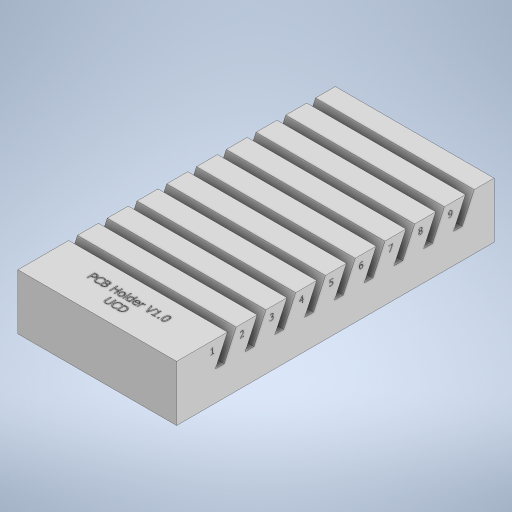
# Autodesk Inventor part: Part1
Saved by Autodesk Inventor 2024 (Build 280153000, 153)
## iProperties
Created: 2024-10-10
Part Number: Part1
Material: Generic
Document SubType Name: Modeling
Designer: Kemper Room 121
Density: 1 g/cm^3
Appearance: Default
Author: Kemper Room 121
Autodesk Inventor part; units mm, degrees
ref_plane "YZ Plane" through (0, 0, 0) normal (1, 0, 0) x (0, 1, 0)
ref_plane "XZ Plane" through (0, 0, 0) normal (0, 1, 0) x (-1, 0, 0)
sketch "Sketch1" plane through (0, 0, 0) normal (1, 0, 0) x (0, 1, 0)
  line L0 (0, 0) -> (10, 0)
  line L1 (10, 0) -> (28, 0)
  line L2 (28, 0) -> (28, -160)
  line L3 (28, -160) -> (0, -160)
  line L4 (0, -160) -> (0, 0)
  dimension "d0" = 10
  dimension "d1" = 18
  dimension "d2" = 160
  constraints: 10 end point, 3 perpendicular, 1 horizontal, 1 point on line
  measures "d0" distance of L0.start L0.end
  measures "d1" distance of L0.end L1.end
  measures "d2" distance of L1.end L2.end
extrude "Extrusion1" add sketch "Sketch1" along normal blind 80
sketch "Sketch2" plane through (80, 0, 0) normal (1, 0, 0) x (0, 0, -1)
  line L0 (0, 28) -> (0, 0) projected
  line L1 (0, 0) -> (0, 5)
  line L2 (160, 0) -> (160, 28) projected
  line L3 (160, 28) -> (0, 28) projected
  line L4 (0, 28) -> (0, 0) projected
  line L5 (0, 0) -> (160, 0) projected
  line L6 (0, 5) -> (160, 5)
  line L7 (160, 5) -> (160, 28)
  line L8 (160, 28) -> (0, 28)
  line L9 (0, 28) -> (0, 5)
  line L10 (160, 28) -> (0, 28) projected
  line L11 (150, 28) -> (139.2749, 5)
  line L12 (145.5865, 28) -> (134.8614, 5)
  line L13 (135, 28) -> (124.2749, 5)
  line L14 (130.5865, 28) -> (119.8614, 5)
  line L15 (120, 28) -> (109.2749, 5)
  line L16 (115.5865, 28) -> (104.8614, 5)
  line L17 (105, 28) -> (94.2749, 5)
  line L18 (100.5865, 28) -> (89.8614, 5)
  line L19 (90, 28) -> (79.2749, 5)
  line L20 (85.5865, 28) -> (74.8614, 5)
  line L21 (75, 28) -> (64.2749, 5)
  line L22 (70.5865, 28) -> (59.8614, 5)
  line L23 (60, 28) -> (49.2749, 5)
  line L24 (55.5865, 28) -> (44.8614, 5)
  line L25 (45, 28) -> (34.2749, 5)
  line L26 (40.5865, 28) -> (29.8614, 5)
  line L27 (30, 28) -> (19.2749, 5)
  line L28 (25.5865, 28) -> (14.8614, 5)
  line L29 (15, 28) -> (4.2749, 5)
  line L30 (10.5865, 28) -> (-0.1386, 5)
  line L31 (10.8067, 29.0831) -> (14.4923, 29.0831) construction
  line L32 (14.4923, 29.0831) -> (14.4923, 25.1764) construction
  line L33 (14.4923, 25.1764) -> (10.8067, 25.1764) construction
  line L34 (10.8067, 25.1764) -> (10.8067, 29.0831) construction
  point P0 (40.5865, 28)
  point P1 (29.8614, 5)
  point P2 (34.2749, 5)
  point P3 (45, 28)
  point P4 (55.5865, 28)
  point P5 (44.8614, 5)
  point P6 (49.2749, 5)
  point P7 (60, 28)
  point P8 (70.5865, 28)
  point P9 (59.8614, 5)
  point P10 (64.2749, 5)
  point P11 (75, 28)
  point P12 (85.5865, 28)
  point P13 (74.8614, 5)
  point P14 (79.2749, 5)
  point P15 (90, 28)
  point P16 (100.5865, 28)
  point P17 (89.8614, 5)
  point P18 (94.2749, 5)
  point P19 (105, 28)
  point P20 (115.5865, 28)
  point P21 (104.8614, 5)
  point P22 (109.2749, 5)
  point P23 (119.8614, 5)
  point P24 (124.2749, 5)
  point P25 (0, 7.2972)
  point P26 (0, 7.2972)
  point P27 (25.5865, 28)
  point P28 (14.8614, 5)
  point P29 (19.2749, 5)
  point P30 (30, 28)
  dimension "d5" = 5
  dimension "d6" = 4
  dimension "d7" = 10
  dimension "d10" = 15
  dimension "d15" = 65
  constraints: 48 end point, 36 horizontal alignment, 20 parallel, 3 point on line, 1 horizontal, 1 vertical, 8 other
  measures "d5" distance of L0.end L1.end
  measures "d6" distance between parallel lines of L12 L11
  measures "d7" distance of L2.end L11.start
  measures "d10" distance of L11.start L13.start
  measures "d15" angle to the sketch x axis of L11
extrude "Extrusion2" cut sketch "Sketch2" against normal through all contours L28 L3 L27 L6 | L6 L12 L3 L11 | L26 L3 L25 L6 | L6 L14 L3 L13 | L24 L3 L23 L6 | L6 L16 L3 L15 | L22 L3 L21 L6 | L6 L18 L3 L17 | L20 L3 L19 L6
sketch "Sketch3" plane through (80, 0, 0) normal (1, 0, 0) x (0, 0, -1)
  line L0 (16.8059, 25) -> (19.0865, 25) construction
  line L1 (19.0865, 25) -> (19.0865, 23.4511) construction
  line L2 (19.0865, 23.4511) -> (16.8059, 23.4511) construction
  line L3 (16.8059, 23.4511) -> (16.8059, 25) construction
  line L4 (31.8059, 25) -> (34.0865, 25) construction
  line L5 (34.0865, 25) -> (34.0865, 23.6664) construction
  line L6 (34.0865, 23.6664) -> (31.8059, 23.6664) construction
  line L7 (31.8059, 23.6664) -> (31.8059, 25) construction
  line L8 (46.8059, 21.9511) -> (46.8059, 25) construction
  line L9 (46.8059, 25) -> (49.0865, 25) construction
  line L10 (49.0865, 25) -> (49.0865, 21.9511) construction
  line L11 (49.0865, 21.9511) -> (46.8059, 21.9511) construction
  line L12 (61.8059, 21.9511) -> (61.8059, 25) construction
  line L13 (61.8059, 25) -> (64.0865, 25) construction
  line L14 (64.0865, 25) -> (64.0865, 21.9511) construction
  line L15 (64.0865, 21.9511) -> (61.8059, 21.9511) construction
  line L16 (76.8059, 21.9511) -> (76.8059, 25) construction
  line L17 (76.8059, 25) -> (79.0865, 25) construction
  line L18 (79.0865, 25) -> (79.0865, 21.9511) construction
  line L19 (79.0865, 21.9511) -> (76.8059, 21.9511) construction
  line L20 (91.8059, 21.9511) -> (91.8059, 25) construction
  line L21 (91.8059, 25) -> (94.0865, 25) construction
  line L22 (94.0865, 25) -> (94.0865, 21.9511) construction
  line L23 (94.0865, 21.9511) -> (91.8059, 21.9511) construction
  line L24 (106.8059, 21.9511) -> (106.8059, 25) construction
  line L25 (106.8059, 25) -> (109.0865, 25) construction
  line L26 (109.0865, 25) -> (109.0865, 21.9511) construction
  line L27 (109.0865, 21.9511) -> (106.8059, 21.9511) construction
  line L28 (121.8059, 21.9511) -> (121.8059, 25) construction
  line L29 (121.8059, 25) -> (124.0865, 25) construction
  line L30 (124.0865, 25) -> (124.0865, 21.9511) construction
  line L31 (124.0865, 21.9511) -> (121.8059, 21.9511) construction
  line L32 (70.5865, 28) -> (0, 28) projected
  line L33 (160, 28) -> (150, 28) projected
  line L34 (70.5865, 28) -> (0, 28) projected
  line L35 (85.5865, 28) -> (75, 28) projected
  line L36 (100.5865, 28) -> (90, 28) projected
  line L37 (115.5865, 28) -> (105, 28) projected
  line L38 (130.5865, 28) -> (120, 28) projected
  line L39 (145.5865, 28) -> (135, 28) projected
  line L40 (0, 28) -> (0, 0) projected
  line L41 (104.8614, 5) -> (115.5865, 28) projected
  line L42 (115.5865, 28) -> (105, 28) projected
  line L43 (105, 28) -> (94.2749, 5) projected
  line L44 (94.2749, 5) -> (89.8614, 5) projected
  line L45 (89.8614, 5) -> (100.5865, 28) projected
  line L46 (100.5865, 28) -> (90, 28) projected
  line L47 (90, 28) -> (79.2749, 5) projected
  line L48 (79.2749, 5) -> (74.8614, 5) projected
  line L49 (74.8614, 5) -> (85.5865, 28) projected
  line L50 (85.5865, 28) -> (75, 28) projected
  line L51 (75, 28) -> (64.2749, 5) projected
  line L52 (64.2749, 5) -> (59.8614, 5) projected
  line L53 (59.8614, 5) -> (70.5865, 28) projected
  line L54 (70.5865, 28) -> (60, 28) projected
  line L55 (60, 28) -> (49.2749, 5) projected
  line L56 (49.2749, 5) -> (44.8614, 5) projected
  line L57 (44.8614, 5) -> (55.5865, 28) projected
  line L58 (55.5865, 28) -> (45, 28) projected
  line L59 (45, 28) -> (34.2749, 5) projected
  line L60 (34.2749, 5) -> (29.8614, 5) projected
  line L61 (29.8614, 5) -> (40.5865, 28) projected
  line L62 (40.5865, 28) -> (30, 28) projected
  line L63 (30, 28) -> (19.2749, 5) projected
  line L64 (19.2749, 5) -> (14.8614, 5) projected
  line L65 (14.8614, 5) -> (25.5865, 28) projected
  line L66 (25.5865, 28) -> (0, 28) projected
  line L67 (0, 28) -> (0, 0) projected
  line L68 (0, 0) -> (160, 0) projected
  line L69 (160, 0) -> (160, 28) projected
  line L70 (160, 28) -> (150, 28) projected
  line L71 (150, 28) -> (139.2749, 5) projected
  line L72 (139.2749, 5) -> (134.8614, 5) projected
  line L73 (134.8614, 5) -> (145.5865, 28) projected
  line L74 (145.5865, 28) -> (135, 28) projected
  line L75 (135, 28) -> (124.2749, 5) projected
  line L76 (124.2749, 5) -> (119.8614, 5) projected
  line L77 (119.8614, 5) -> (130.5865, 28) projected
  line L78 (130.5865, 28) -> (120, 28) projected
  line L79 (120, 28) -> (109.2749, 5) projected
  line L80 (109.2749, 5) -> (104.8614, 5) projected
  line L81 (136.8059, 21.9511) -> (136.8059, 25) construction
  line L82 (136.8059, 25) -> (139.0865, 25) construction
  line L83 (139.0865, 25) -> (139.0865, 21.9511) construction
  line L84 (139.0865, 21.9511) -> (136.8059, 21.9511) construction
  line L85 (18.7548, 21.9421) -> (17.2678, 21.9421)
  line L86 (17.2678, 21.9421) -> (17.2678, 22.2533)
  line L87 (17.2678, 22.2533) -> (17.8211, 22.2533)
  line L88 (17.8211, 22.2533) -> (17.8211, 24.296)
  line L89 (17.8211, 24.296) -> (17.2678, 24.296)
  line L90 (17.2678, 24.296) -> (17.2678, 24.5752)
  spline S0 degree 2 poles (17.2678, 24.5752) (17.5815, 24.5752) (17.8779, 24.753) (17.8977, 25) knots 0 0 0 1 2 2 2
  line L91 (17.8977, 25) -> (18.2139, 25)
  line L92 (18.2139, 25) -> (18.2139, 22.2533)
  line L93 (18.2139, 22.2533) -> (18.7548, 22.2533)
  line L94 (18.7548, 22.2533) -> (18.7548, 21.9421)
  line L95 (33.9079, 21.8878) -> (32.0282, 21.8878)
  line L96 (32.0282, 21.8878) -> (32.0282, 22.32)
  spline S1 degree 2 poles (32.0282, 22.32) (32.2308, 22.5102) (32.5914, 22.8634) (32.7643, 23.0536) knots 0 0 0 1 2 2 2
  spline S2 degree 2 poles (32.7643, 23.0536) (33.1126, 23.4365) (33.367, 23.8959) (33.367, 24.1404) knots 0 0 0 1 2 2 2
  spline S3 degree 2 poles (33.367, 24.1404) (33.367, 24.2689) (33.288, 24.4615) (33.2163, 24.5233) knots 0 0 0 1 2 2 2
  spline S4 degree 2 poles (33.2163, 24.5233) (33.1447, 24.585) (32.957, 24.6468) (32.8434, 24.6468) knots 0 0 0 1 2 2 2
  spline S5 degree 2 poles (32.8434, 24.6468) (32.7347, 24.6468) (32.5124, 24.5924) (32.4111, 24.5505) knots 0 0 0 1 2 2 2
  spline S6 degree 2 poles (32.4111, 24.5505) (32.3247, 24.5159) (32.1641, 24.4171) (32.1147, 24.3825) knots 0 0 0 1 2 2 2
  line L97 (32.1147, 24.3825) -> (32.0925, 24.3825)
  line L98 (32.0925, 24.3825) -> (32.0925, 24.8172)
  spline S7 degree 2 poles (32.0925, 24.8172) (32.2184, 24.879) (32.6705, 25) (32.873, 25) knots 0 0 0 1 2 2 2
  spline S8 degree 2 poles (32.873, 25) (33.3003, 25) (33.782, 24.548) (33.782, 24.1627) knots 0 0 0 1 2 2 2
  spline S9 degree 2 poles (33.782, 24.1627) (33.782, 23.9824) (33.698, 23.681) (33.6239, 23.5526) knots 0 0 0 1 2 2 2
  spline S10 degree 2 poles (33.6239, 23.5526) (33.5498, 23.4192) (33.3349, 23.1574) (33.2163, 23.0314) knots 0 0 0 1 2 2 2
  spline S11 degree 2 poles (33.2163, 23.0314) (33.0237, 22.8214) (32.5519, 22.3719) (32.4111, 22.241) knots 0 0 0 1 2 2 2
  line L99 (32.4111, 22.241) -> (33.9079, 22.241)
  line L100 (33.9079, 22.241) -> (33.9079, 21.8878)
  spline S12 degree 2 poles (47.8508, 24.6468) (47.7396, 24.6468) (47.5198, 24.5924) (47.4136, 24.5505) knots 0 0 0 1 2 2 2
  spline S13 degree 2 poles (47.4136, 24.5505) (47.3148, 24.5085) (47.169, 24.4195) (47.1122, 24.38) knots 0 0 0 1 2 2 2
  line L101 (47.1122, 24.38) -> (47.0875, 24.38)
  line L102 (47.0875, 24.38) -> (47.0875, 24.8123)
  spline S14 degree 2 poles (47.0875, 24.8123) (47.2209, 24.8839) (47.6779, 25) (47.8829, 25) knots 0 0 0 1 2 2 2
  spline S15 degree 2 poles (47.8829, 25) (48.0904, 25) (48.3991, 24.916) (48.5251, 24.8271) knots 0 0 0 1 2 2 2
  spline S16 degree 2 poles (48.5251, 24.8271) (48.6585, 24.7308) (48.7968, 24.4517) (48.7968, 24.2639) knots 0 0 0 1 2 2 2
  spline S17 degree 2 poles (48.7968, 24.2639) (48.7968, 24.012) (48.4658, 23.6316) (48.2336, 23.5822) knots 0 0 0 1 2 2 2
  line L103 (48.2336, 23.5822) -> (48.2336, 23.5526)
  spline S18 degree 2 poles (48.2336, 23.5526) (48.3299, 23.5328) (48.5498, 23.4439) (48.6436, 23.355) knots 0 0 0 1 2 2 2
  spline S19 degree 2 poles (48.6436, 23.355) (48.7375, 23.2685) (48.8561, 22.9919) (48.8561, 22.7918) knots 0 0 0 1 2 2 2
  spline S20 degree 2 poles (48.8561, 22.7918) (48.8561, 22.5868) (48.7153, 22.2385) (48.5868, 22.1051) knots 0 0 0 1 2 2 2
  spline S21 degree 2 poles (48.5868, 22.1051) (48.4534, 21.9668) (48.0755, 21.8236) (47.8359, 21.8236) knots 0 0 0 1 2 2 2
  spline S22 degree 2 poles (47.8359, 21.8236) (47.6062, 21.8236) (47.1567, 21.9347) (47.0035, 22.0113) knots 0 0 0 1 2 2 2
  line L104 (47.0035, 22.0113) -> (47.0035, 22.4435)
  line L105 (47.0035, 22.4435) -> (47.0332, 22.4435)
  spline S23 degree 2 poles (47.0332, 22.4435) (47.1616, 22.3497) (47.5964, 22.1768) (47.8112, 22.1768) knots 0 0 0 1 2 2 2
  spline S24 degree 2 poles (47.8112, 22.1768) (47.9372, 22.1768) (48.1892, 22.2558) (48.2731, 22.3472) knots 0 0 0 1 2 2 2
  spline S25 degree 2 poles (48.2731, 22.3472) (48.3546, 22.4386) (48.4411, 22.656) (48.4411, 22.8214) knots 0 0 0 1 2 2 2
  spline S26 degree 2 poles (48.4411, 22.8214) (48.4411, 22.9869) (48.3448, 23.2018) (48.2583, 23.2636) knots 0 0 0 1 2 2 2
  spline S27 degree 2 poles (48.2583, 23.2636) (48.1719, 23.3253) (47.9372, 23.3723) (47.7989, 23.3723) knots 0 0 0 1 2 2 2
  line L106 (47.7989, 23.3723) -> (47.626, 23.3723)
  line L107 (47.626, 23.3723) -> (47.626, 23.7107)
  line L108 (47.626, 23.7107) -> (47.7618, 23.7107)
  spline S28 degree 2 poles (47.7618, 23.7107) (48.036, 23.7107) (48.3818, 23.9725) (48.3818, 24.2219) knots 0 0 0 1 2 2 2
  spline S29 degree 2 poles (48.3818, 24.2219) (48.3818, 24.338) (48.2929, 24.5035) (48.2213, 24.5529) knots 0 0 0 1 2 2 2
  spline S30 degree 2 poles (48.2213, 24.5529) (48.1447, 24.6048) (47.957, 24.6468) (47.8508, 24.6468) knots 0 0 0 1 2 2 2
  line L109 (63.9894, 22.9993) -> (63.6263, 22.9993)
  line L110 (63.6263, 22.9993) -> (63.6263, 21.952)
  line L111 (63.6263, 21.952) -> (63.2336, 21.952)
  line L112 (63.2336, 21.952) -> (63.2336, 22.9993)
  line L113 (63.2336, 22.9993) -> (61.8875, 22.9993)
  line L114 (61.8875, 22.9993) -> (61.8875, 23.4291)
  line L115 (61.8875, 23.4291) -> (63.2509, 25)
  line L116 (63.2509, 25) -> (63.6263, 25)
  line L117 (63.6263, 25) -> (63.6263, 23.3278)
  line L118 (63.6263, 23.3278) -> (63.9894, 23.3278)
  line L119 (63.9894, 23.3278) -> (63.9894, 22.9993)
  line L120 (63.2336, 23.3278) -> (63.2336, 24.5183)
  line L121 (63.2336, 24.5183) -> (62.2086, 23.3278)
  line L122 (62.2086, 23.3278) -> (63.2336, 23.3278)
  spline S31 degree 2 poles (78.8758, 22.9202) (78.8758, 22.7004) (78.735, 22.325) (78.6066, 22.1867) knots 0 0 0 1 2 2 2
  spline S32 degree 2 poles (78.6066, 22.1867) (78.4781, 22.0483) (78.0953, 21.8878) (77.8582, 21.8878) knots 0 0 0 1 2 2 2
  spline S33 degree 2 poles (77.8582, 21.8878) (77.6408, 21.8878) (77.216, 21.9841) (77.0604, 22.0607) knots 0 0 0 1 2 2 2
  line L123 (77.0604, 22.0607) -> (77.0604, 22.4929)
  line L124 (77.0604, 22.4929) -> (77.09, 22.4929)
  spline S34 degree 2 poles (77.09, 22.4929) (77.1369, 22.4584) (77.3123, 22.3694) (77.4185, 22.3299) knots 0 0 0 1 2 2 2
  spline S35 degree 2 poles (77.4185, 22.3299) (77.5395, 22.2879) (77.7396, 22.241) (77.8656, 22.241) knots 0 0 0 1 2 2 2
  spline S36 degree 2 poles (77.8656, 22.241) (77.9891, 22.241) (78.2213, 22.3299) (78.3052, 22.4262) knots 0 0 0 1 2 2 2
  spline S37 degree 2 poles (78.3052, 22.4262) (78.3818, 22.5176) (78.4609, 22.7597) (78.4609, 22.9227) knots 0 0 0 1 2 2 2
  spline S38 degree 2 poles (78.4609, 22.9227) (78.4609, 23.0857) (78.3719, 23.2932) (78.288, 23.3624) knots 0 0 0 1 2 2 2
  spline S39 degree 2 poles (78.288, 23.3624) (78.2015, 23.4389) (77.9446, 23.5032) (77.789, 23.5032) knots 0 0 0 1 2 2 2
  spline S40 degree 2 poles (77.789, 23.5032) (77.6211, 23.5032) (77.2876, 23.4513) (77.1863, 23.4291) knots 0 0 0 1 2 2 2
  line L125 (77.1863, 23.4291) -> (77.1863, 25)
  line L126 (77.1863, 25) -> (78.8585, 25)
  line L127 (78.8585, 25) -> (78.8585, 24.6418)
  line L128 (78.8585, 24.6418) -> (77.5791, 24.6418)
  line L129 (77.5791, 24.6418) -> (77.5791, 23.8292)
  spline S41 degree 2 poles (77.5791, 23.8292) (77.6532, 23.8391) (77.7964, 23.8465) (77.8557, 23.8465) knots 0 0 0 1 2 2 2
  spline S42 degree 2 poles (77.8557, 23.8465) (78.0904, 23.8465) (78.4139, 23.7699) (78.5621, 23.6563) knots 0 0 0 1 2 2 2
  spline S43 degree 2 poles (78.5621, 23.6563) (78.7128, 23.5427) (78.8758, 23.1969) (78.8758, 22.9202) knots 0 0 0 1 2 2 2
  spline S44 degree 2 poles (93.9549, 22.8832) (93.9549, 22.6485) (93.7993, 22.2509) (93.6683, 22.1175) knots 0 0 0 1 2 2 2
  spline S45 degree 2 poles (93.6683, 22.1175) (93.5325, 21.9767) (93.1916, 21.831) (92.9866, 21.831) knots 0 0 0 1 2 2 2
  spline S46 degree 2 poles (92.9866, 21.831) (92.7816, 21.831) (92.4432, 21.9693) (92.3148, 22.1076) knots 0 0 0 1 2 2 2
  spline S47 degree 2 poles (92.3148, 22.1076) (92.1567, 22.2731) (91.9788, 22.8289) (91.9788, 23.2339) knots 0 0 0 1 2 2 2
  spline S48 degree 2 poles (91.9788, 23.2339) (91.9788, 23.6316) (92.1419, 24.2713) (92.3123, 24.5085) knots 0 0 0 1 2 2 2
  spline S49 degree 2 poles (92.3123, 24.5085) (92.4778, 24.7406) (93.0014, 25) (93.3448, 25) knots 0 0 0 1 2 2 2
  spline S50 degree 2 poles (93.3448, 25) (93.446, 25) (93.6239, 24.9802) (93.6906, 24.958) knots 0 0 0 1 2 2 2
  line L130 (93.6906, 24.958) -> (93.6906, 24.5653)
  line L131 (93.6906, 24.5653) -> (93.6733, 24.5653)
  spline S51 degree 2 poles (93.6733, 24.5653) (93.6165, 24.5949) (93.409, 24.6468) (93.2904, 24.6468) knots 0 0 0 1 2 2 2
  spline S52 degree 2 poles (93.2904, 24.6468) (92.91, 24.6468) (92.4432, 24.133) (92.3988, 23.6291) knots 0 0 0 1 2 2 2
  spline S53 degree 2 poles (92.3988, 23.6291) (92.5445, 23.7304) (92.8508, 23.8416) (93.0335, 23.8416) knots 0 0 0 1 2 2 2
  spline S54 degree 2 poles (93.0335, 23.8416) (93.2114, 23.8416) (93.4781, 23.7699) (93.6239, 23.6613) knots 0 0 0 1 2 2 2
  spline S55 degree 2 poles (93.6239, 23.6613) (93.7918, 23.5353) (93.9549, 23.145) (93.9549, 22.8832) knots 0 0 0 1 2 2 2
  spline S56 degree 2 poles (93.5399, 22.8659) (93.5399, 23.0536) (93.4411, 23.308) (93.3324, 23.397) knots 0 0 0 1 2 2 2
  spline S57 degree 2 poles (93.3324, 23.397) (93.2509, 23.4612) (93.0484, 23.5032) (92.9422, 23.5032) knots 0 0 0 1 2 2 2
  spline S58 degree 2 poles (92.9422, 23.5032) (92.7989, 23.5032) (92.5297, 23.4167) (92.3988, 23.3352) knots 0 0 0 1 2 2 2
  spline S59 degree 2 poles (92.3988, 23.3352) (92.3963, 23.2907) (92.3913, 23.2068) (92.3913, 23.1425) knots 0 0 0 1 2 2 2
  spline S60 degree 2 poles (92.3913, 23.1425) (92.3913, 22.8264) (92.5148, 22.4386) (92.6087, 22.3373) knots 0 0 0 1 2 2 2
  spline S61 degree 2 poles (92.6087, 22.3373) (92.6952, 22.241) (92.8829, 22.1644) (92.9891, 22.1644) knots 0 0 0 1 2 2 2
  spline S62 degree 2 poles (92.9891, 22.1644) (93.2361, 22.1644) (93.5399, 22.5152) (93.5399, 22.8659) knots 0 0 0 1 2 2 2
  line L132 (108.9425, 24.543) -> (107.6235, 21.952)
  line L133 (107.6235, 21.952) -> (107.1888, 21.952)
  line L134 (107.1888, 21.952) -> (108.5819, 24.6418)
  line L135 (108.5819, 24.6418) -> (107.0085, 24.6418)
  line L136 (107.0085, 24.6418) -> (107.0085, 25)
  line L137 (107.0085, 25) -> (108.9425, 25)
  line L138 (108.9425, 25) -> (108.9425, 24.543)
  spline S63 degree 2 poles (122.9496, 21.8137) (122.7223, 21.8137) (122.3494, 21.9495) (122.2184, 22.0755) knots 0 0 0 1 2 2 2
  spline S64 degree 2 poles (122.2184, 22.0755) (122.09, 22.199) (121.9566, 22.5349) (121.9566, 22.7251) knots 0 0 0 1 2 2 2
  spline S65 degree 2 poles (121.9566, 22.7251) (121.9566, 22.9721) (122.2209, 23.3871) (122.4729, 23.5106) knots 0 0 0 1 2 2 2
  line L139 (122.4729, 23.5106) -> (122.4729, 23.5229)
  spline S66 degree 2 poles (122.4729, 23.5229) (122.2481, 23.6538) (122.0307, 23.9651) (122.0307, 24.1972) knots 0 0 0 1 2 2 2
  spline S67 degree 2 poles (122.0307, 24.1972) (122.0307, 24.5406) (122.5494, 25) (122.9496, 25) knots 0 0 0 1 2 2 2
  spline S68 degree 2 poles (122.9496, 25) (123.3645, 25) (123.8659, 24.5653) (123.8659, 24.2244) knots 0 0 0 1 2 2 2
  spline S69 degree 2 poles (123.8659, 24.2244) (123.8659, 24.0194) (123.6263, 23.6193) (123.4016, 23.5056) knots 0 0 0 1 2 2 2
  line L140 (123.4016, 23.5056) -> (123.4016, 23.4933)
  spline S70 degree 2 poles (123.4016, 23.4933) (123.6683, 23.3698) (123.9425, 23.0141) (123.9425, 22.7325) knots 0 0 0 1 2 2 2
  spline S71 degree 2 poles (123.9425, 22.7325) (123.9425, 22.3423) (123.3744, 21.8137) (122.9496, 21.8137) knots 0 0 0 1 2 2 2
  spline S72 degree 2 poles (123.5226, 22.693) (123.5226, 22.8807) (123.3744, 23.103) (123.1645, 23.2166) knots 0 0 0 1 2 2 2
  spline S73 degree 2 poles (123.1645, 23.2166) (123.0953, 23.2562) (122.8631, 23.3476) (122.7174, 23.4068) knots 0 0 0 1 2 2 2
  spline S74 degree 2 poles (122.7174, 23.4068) (122.5494, 23.2957) (122.3691, 22.9647) (122.3691, 22.7548) knots 0 0 0 1 2 2 2
  spline S75 degree 2 poles (122.3691, 22.7548) (122.3691, 22.4781) (122.7026, 22.1175) (122.9545, 22.1175) knots 0 0 0 1 2 2 2
  spline S76 degree 2 poles (122.9545, 22.1175) (123.2114, 22.1175) (123.5226, 22.4262) (123.5226, 22.693) knots 0 0 0 1 2 2 2
  spline S77 degree 2 poles (123.4658, 24.2195) (123.4658, 24.4245) (123.1916, 24.6987) (122.9471, 24.6987) knots 0 0 0 1 2 2 2
  spline S78 degree 2 poles (122.9471, 24.6987) (122.7248, 24.6987) (122.4407, 24.4541) (122.4407, 24.2442) knots 0 0 0 1 2 2 2
  spline S79 degree 2 poles (122.4407, 24.2442) (122.4407, 24.0935) (122.5865, 23.8836) (122.7322, 23.7996) knots 0 0 0 1 2 2 2
  spline S80 degree 2 poles (122.7322, 23.7996) (122.794, 23.765) (123.0558, 23.644) (123.162, 23.6094) knots 0 0 0 1 2 2 2
  spline S81 degree 2 poles (123.162, 23.6094) (123.3398, 23.7452) (123.4658, 24.0342) (123.4658, 24.2195) knots 0 0 0 1 2 2 2
  spline S82 degree 2 poles (136.9443, 23.9478) (136.9443, 24.1824) (137.0974, 24.5727) (137.2308, 24.7135) knots 0 0 0 1 2 2 2
  spline S83 degree 2 poles (137.2308, 24.7135) (137.3568, 24.8493) (137.7248, 25) (137.9125, 25) knots 0 0 0 1 2 2 2
  spline S84 degree 2 poles (137.9125, 25) (138.1225, 25) (138.4633, 24.8592) (138.5893, 24.7258) knots 0 0 0 1 2 2 2
  spline S85 degree 2 poles (138.5893, 24.7258) (138.7474, 24.5579) (138.9203, 24.0145) (138.9203, 23.597) knots 0 0 0 1 2 2 2
  spline S86 degree 2 poles (138.9203, 23.597) (138.9203, 23.2191) (138.7499, 22.5423) (138.5844, 22.3176) knots 0 0 0 1 2 2 2
  spline S87 degree 2 poles (138.5844, 22.3176) (138.409, 22.0804) (137.915, 21.831) (137.5544, 21.831) knots 0 0 0 1 2 2 2
  spline S88 degree 2 poles (137.5544, 21.831) (137.4729, 21.831) (137.2876, 21.8483) (137.2086, 21.873) knots 0 0 0 1 2 2 2
  line L141 (137.2086, 21.873) -> (137.2086, 22.2657)
  line L142 (137.2086, 22.2657) -> (137.2283, 22.2657)
  spline S89 degree 2 poles (137.2283, 22.2657) (137.2802, 22.2361) (137.4976, 22.1842) (137.6087, 22.1842) knots 0 0 0 1 2 2 2
  spline S90 degree 2 poles (137.6087, 22.1842) (138.0088, 22.1842) (138.4658, 22.7128) (138.4979, 23.2018) knots 0 0 0 1 2 2 2
  spline S91 degree 2 poles (138.4979, 23.2018) (138.3349, 23.0907) (138.0385, 22.9894) (137.8631, 22.9894) knots 0 0 0 1 2 2 2
  spline S92 degree 2 poles (137.8631, 22.9894) (137.6952, 22.9894) (137.416, 23.0635) (137.2753, 23.1697) knots 0 0 0 1 2 2 2
  spline S93 degree 2 poles (137.2753, 23.1697) (137.1122, 23.2957) (136.9443, 23.6785) (136.9443, 23.9478) knots 0 0 0 1 2 2 2
  spline S94 degree 2 poles (138.5078, 23.6884) (138.5078, 23.9972) (138.3942, 24.3874) (138.2929, 24.4936) knots 0 0 0 1 2 2 2
  spline S95 degree 2 poles (138.2929, 24.4936) (138.204, 24.5924) (138.0187, 24.6665) (137.91, 24.6665) knots 0 0 0 1 2 2 2
  spline S96 degree 2 poles (137.91, 24.6665) (137.6581, 24.6665) (137.3592, 24.3059) (137.3592, 23.9651) knots 0 0 0 1 2 2 2
  spline S97 degree 2 poles (137.3592, 23.9651) (137.3592, 23.7724) (137.458, 23.5229) (137.5667, 23.434) knots 0 0 0 1 2 2 2
  spline S98 degree 2 poles (137.5667, 23.434) (137.6458, 23.3698) (137.8409, 23.3278) (137.9545, 23.3278) knots 0 0 0 1 2 2 2
  spline S99 degree 2 poles (137.9545, 23.3278) (138.0854, 23.3278) (138.3868, 23.4192) (138.5004, 23.4958) knots 0 0 0 1 2 2 2
  spline S100 degree 2 poles (138.5004, 23.4958) (138.5028, 23.5254) (138.5078, 23.6267) (138.5078, 23.6884) knots 0 0 0 1 2 2 2
  point P0 (17.9462, 23.4511)
  point P1 (32.9462, 23.6664)
  point P2 (47.9462, 21.9511)
  point P3 (62.9462, 21.9511)
  point P4 (77.9462, 21.9511)
  point P5 (92.9462, 21.9511)
  point P6 (107.9462, 21.9511)
  point P7 (122.9462, 21.9511)
  point P8 (47.9462, 25)
  point P9 (32.9462, 25)
  point P10 (62.9462, 25)
  point P11 (77.9462, 25)
  point P12 (92.9462, 25)
  point P13 (107.9462, 25)
  point P14 (122.9462, 25)
  point P15 (137.9462, 21.9511)
  point P16 (137.9462, 25)
  dimension "d23" = 15
  dimension "d24" = 3
  dimension "d25" = 15
  dimension "d26" = 15
  dimension "d27" = 15
  dimension "d28" = 15
  dimension "d29" = 15
  dimension "d30" = 15
  dimension "d31" = 3
  dimension "d32" = 3
  dimension "d33" = 3
  dimension "d34" = 3
  dimension "d35" = 3
  dimension "d36" = 3
  dimension "d37" = 3
  dimension "d38" = 2.2805
  dimension "d41" = 6.5
  dimension "d42" = 15
  dimension "d43" = 3
  constraints: 17 midpoint, 18 other
  measures "d23" horizontal distance of point (17.946, 23.451) point (32.946, 23.666)
  measures "d24" distance between parallel lines of L32 L0
  measures "d25" distance of point (47.946, 25) point (32.946, 25)
  measures "d26" distance of point (62.946, 25) point (47.946, 25)
  measures "d27" distance of point (77.946, 25) point (62.946, 25)
  measures "d28" distance of point (92.946, 25) point (77.946, 25)
  measures "d29" distance of point (107.946, 25) point (92.946, 25)
  measures "d30" distance of point (122.946, 25) point (107.946, 25)
  measures "d31" distance from line of L33 point (32.946, 25)
  measures "d32" distance from line of L34 point (47.946, 25)
  measures "d33" distance from line of L35 point (62.946, 25)
  measures "d34" distance from line of L36 point (77.946, 25)
  measures "d35" distance from line of L37 point (92.946, 25)
  measures "d36" distance from line of L38 point (107.946, 25)
  measures "d37" distance from line of L39 point (122.946, 25)
  measures "d38" distance of L5.end L7.start
  measures "d41" distance from line of L65.end L1
  measures "d42" distance of point (137.946, 25) point (122.946, 25)
  measures "d43" distance between parallel lines of L39 L82
emboss "Emboss1" sketch "Sketch3" operation cut depth 5 direction (-1, 0, 0) contours L85 L86 L87 L88 L89 L90 S0 L91 L92 L93 L94 | L95 L96 S1 S2 S3 S4 S5 S6 L97 L98 S7 S8 S9 S10 S11 L99 L100 | S12 S13 L101 L102 S14 S15 S16 S17 L103 S18 S19 S20 S21 S22 L104 L105 S23 S24 S25 S26 S27 L106 L107 L108 S28 S29 S30 | L109 L110 L111 L112 L113 L114 L115 L116 L117 L118 L119 | S31 S32 S33 L123 L124 S34 S35 S36 S37 S38 S39 S40 L125 L126 L127 L128 L129 S41 S42 S43 | S44 S45 S46 S47 S48 S49 S50 L130 L131 S51 S52 S53 S54 S55 | L132 L133 L134 L135 L136 L137 L138 | S63 S64 S65 L139 S66 S67 S68 S69 L140 S70 S71 | S82 S83 S84 S85 S86 S87 S88 L141 L142 S89 S90 S91 S92 S93
sketch "Sketch4" plane through (0, 28, 0) normal (0, 1, 0) x (1, 0, 0)
  line L0 (80, 25.5865) -> (0, 25.5865) projected
  line L1 (0, 25.5865) -> (0, 0) projected
  line L2 (0, 0) -> (80, 0) projected
  line L3 (80, 25.5865) -> (80, 0) projected
  line L4 (0.5027, 25.1634) -> (79.9363, 25.1634) construction
  line L5 (79.9363, 25.1634) -> (79.9363, 0.3404) construction
  line L6 (79.9363, 0.3404) -> (0.5027, 0.3404) construction
  line L7 (0.5027, 0.3404) -> (0.5027, 25.1634) construction
  spline S0 degree 2 poles (23.2308, 16.792) (23.2308, 16.5327) (23.0461, 16.0659) (22.8808, 15.9038) knots 0 0 0 1 2 2 2
  spline S1 degree 2 poles (22.8808, 15.9038) (22.6733, 15.6996) (22.1125, 15.4889) (21.6846, 15.4889) knots 0 0 0 1 2 2 2
  line L8 (21.6846, 15.4889) -> (21.2341, 15.4889)
  line L9 (21.2341, 15.4889) -> (21.2341, 13.9978)
  line L10 (21.2341, 13.9978) -> (20.7025, 13.9978)
  line L11 (20.7025, 13.9978) -> (20.7025, 17.9978)
  line L12 (20.7025, 17.9978) -> (21.7073, 17.9978)
  spline S2 degree 2 poles (21.7073, 17.9978) (22.0639, 17.9978) (22.5631, 17.8811) (22.7543, 17.7482) knots 0 0 0 1 2 2 2
  spline S3 degree 2 poles (22.7543, 17.7482) (22.978, 17.5959) (23.2308, 17.1258) (23.2308, 16.792) knots 0 0 0 1 2 2 2
  spline S4 degree 2 poles (22.6765, 16.7758) (22.6765, 16.9832) (22.5339, 17.2879) (22.388, 17.3852) knots 0 0 0 1 2 2 2
  spline S5 degree 2 poles (22.388, 17.3852) (22.2616, 17.4694) (21.9245, 17.5375) (21.6749, 17.5375) knots 0 0 0 1 2 2 2
  line L13 (21.6749, 17.5375) -> (21.2341, 17.5375)
  line L14 (21.2341, 17.5375) -> (21.2341, 15.9427)
  line L15 (21.2341, 15.9427) -> (21.5971, 15.9427)
  spline S6 degree 2 poles (21.5971, 15.9427) (21.9213, 15.9427) (22.32, 16.0464) (22.4496, 16.1826) knots 0 0 0 1 2 2 2
  spline S7 degree 2 poles (22.4496, 16.1826) (22.5696, 16.3025) (22.6765, 16.5845) (22.6765, 16.7758) knots 0 0 0 1 2 2 2
  spline S8 degree 2 poles (25.2989, 13.9265) (24.9099, 13.9265) (24.2519, 14.1891) (24.012, 14.4516) knots 0 0 0 1 2 2 2
  spline S9 degree 2 poles (24.012, 14.4516) (23.7722, 14.7109) (23.5096, 15.4889) (23.5096, 15.9946) knots 0 0 0 1 2 2 2
  spline S10 degree 2 poles (23.5096, 15.9946) (23.5096, 16.497) (23.7657, 17.2425) (24.0088, 17.5181) knots 0 0 0 1 2 2 2
  spline S11 degree 2 poles (24.0088, 17.5181) (24.2487, 17.7871) (24.9034, 18.0691) (25.3086, 18.0691) knots 0 0 0 1 2 2 2
  spline S12 degree 2 poles (25.3086, 18.0691) (25.5096, 18.0691) (25.8629, 18.0108) (26.012, 17.9654) knots 0 0 0 1 2 2 2
  spline S13 degree 2 poles (26.012, 17.9654) (26.1417, 17.9233) (26.4107, 17.8033) (26.5436, 17.732) knots 0 0 0 1 2 2 2
  line L16 (26.5436, 17.732) -> (26.5436, 17.0902)
  line L17 (26.5436, 17.0902) -> (26.5015, 17.0902)
  spline S14 degree 2 poles (26.5015, 17.0902) (26.4302, 17.155) (26.2098, 17.3365) (26.0509, 17.4241) knots 0 0 0 1 2 2 2
  spline S15 degree 2 poles (26.0509, 17.4241) (25.8986, 17.5083) (25.5388, 17.6153) (25.3054, 17.6153) knots 0 0 0 1 2 2 2
  spline S16 degree 2 poles (25.3054, 17.6153) (25.0493, 17.6153) (24.5923, 17.4046) (24.4205, 17.2036) knots 0 0 0 1 2 2 2
  spline S17 degree 2 poles (24.4205, 17.2036) (24.2519, 16.9994) (24.0639, 16.3803) (24.0639, 15.9946) knots 0 0 0 1 2 2 2
  spline S18 degree 2 poles (24.0639, 15.9946) (24.0639, 15.5829) (24.2616, 14.9897) (24.4334, 14.7855) knots 0 0 0 1 2 2 2
  spline S19 degree 2 poles (24.4334, 14.7855) (24.602, 14.5878) (25.0526, 14.3868) (25.3054, 14.3868) knots 0 0 0 1 2 2 2
  spline S20 degree 2 poles (25.3054, 14.3868) (25.5355, 14.3868) (25.9278, 14.5002) (26.0801, 14.5845) knots 0 0 0 1 2 2 2
  spline S21 degree 2 poles (26.0801, 14.5845) (26.226, 14.6688) (26.4431, 14.8438) (26.5047, 14.9054) knots 0 0 0 1 2 2 2
  line L18 (26.5047, 14.9054) -> (26.5436, 14.9054)
  line L19 (26.5436, 14.9054) -> (26.5436, 14.2701)
  spline S22 degree 2 poles (26.5436, 14.2701) (26.4107, 14.2085) (26.1773, 14.0951) (26.012, 14.0432) knots 0 0 0 1 2 2 2
  spline S23 degree 2 poles (26.012, 14.0432) (25.837, 13.9848) (25.5388, 13.9265) (25.2989, 13.9265) knots 0 0 0 1 2 2 2
  spline S24 degree 2 poles (29.7527, 15.2263) (29.7527, 14.9281) (29.5258, 14.4711) (29.3378, 14.322) knots 0 0 0 1 2 2 2
  spline S25 degree 2 poles (29.3378, 14.322) (29.1109, 14.1469) (28.5955, 13.9978) (28.1871, 13.9978) knots 0 0 0 1 2 2 2
  line L20 (28.1871, 13.9978) -> (27.0396, 13.9978)
  line L21 (27.0396, 13.9978) -> (27.0396, 17.9978)
  line L22 (27.0396, 17.9978) -> (28.0996, 17.9978)
  spline S26 degree 2 poles (28.0996, 17.9978) (28.5274, 17.9978) (28.9553, 17.9427) (29.1498, 17.8357) knots 0 0 0 1 2 2 2
  spline S27 degree 2 poles (29.1498, 17.8357) (29.367, 17.7223) (29.5647, 17.3495) (29.5647, 17.0967) knots 0 0 0 1 2 2 2
  spline S28 degree 2 poles (29.5647, 17.0967) (29.5647, 16.8147) (29.2665, 16.3673) (29.0039, 16.2409) knots 0 0 0 1 2 2 2
  line L23 (29.0039, 16.2409) -> (29.0039, 16.2215)
  spline S29 degree 2 poles (29.0039, 16.2215) (29.3605, 16.1242) (29.7527, 15.6088) (29.7527, 15.2263) knots 0 0 0 1 2 2 2
  spline S30 degree 2 poles (29.1984, 15.2036) (29.1984, 15.4305) (29.0688, 15.7223) (28.8743, 15.826) knots 0 0 0 1 2 2 2
  spline S31 degree 2 poles (28.8743, 15.826) (28.7478, 15.8908) (28.4496, 15.9297) (28.1741, 15.9297) knots 0 0 0 1 2 2 2
  line L24 (28.1741, 15.9297) -> (27.5712, 15.9297)
  line L25 (27.5712, 15.9297) -> (27.5712, 14.4516)
  line L26 (27.5712, 14.4516) -> (28.0023, 14.4516)
  spline S32 degree 2 poles (28.0023, 14.4516) (28.3524, 14.4516) (28.7543, 14.5164) (28.9099, 14.6202) knots 0 0 0 1 2 2 2
  spline S33 degree 2 poles (28.9099, 14.6202) (29.059, 14.7271) (29.1984, 14.9929) (29.1984, 15.2036) knots 0 0 0 1 2 2 2
  spline S34 degree 2 poles (29.0104, 17.0221) (29.0104, 17.1647) (28.9132, 17.3787) (28.8062, 17.4403) knots 0 0 0 1 2 2 2
  spline S35 degree 2 poles (28.8062, 17.4403) (28.6765, 17.5116) (28.3621, 17.544) (28.0801, 17.544) knots 0 0 0 1 2 2 2
  line L27 (28.0801, 17.544) -> (27.5712, 17.544)
  line L28 (27.5712, 17.544) -> (27.5712, 16.3738)
  line L29 (27.5712, 16.3738) -> (28.1741, 16.3738)
  spline S36 degree 2 poles (28.1741, 16.3738) (28.4237, 16.3738) (28.6603, 16.4257) (28.7867, 16.5067) knots 0 0 0 1 2 2 2
  spline S37 degree 2 poles (28.7867, 16.5067) (28.9099, 16.5845) (29.0104, 16.8341) (29.0104, 17.0221) knots 0 0 0 1 2 2 2
  line L30 (34.9034, 13.9978) -> (34.3718, 13.9978)
  line L31 (34.3718, 13.9978) -> (34.3718, 15.9557)
  line L32 (34.3718, 15.9557) -> (32.5307, 15.9557)
  line L33 (32.5307, 15.9557) -> (32.5307, 13.9978)
  line L34 (32.5307, 13.9978) -> (31.9991, 13.9978)
  line L35 (31.9991, 13.9978) -> (31.9991, 17.9978)
  line L36 (31.9991, 17.9978) -> (32.5307, 17.9978)
  line L37 (32.5307, 17.9978) -> (32.5307, 16.4289)
  line L38 (32.5307, 16.4289) -> (34.3718, 16.4289)
  line L39 (34.3718, 16.4289) -> (34.3718, 17.9978)
  line L40 (34.3718, 17.9978) -> (34.9034, 17.9978)
  line L41 (34.9034, 17.9978) -> (34.9034, 13.9978)
  spline S38 degree 2 poles (38.1417, 15.4986) (38.1417, 14.7401) (37.4124, 13.9135) (36.803, 13.9135) knots 0 0 0 1 2 2 2
  spline S39 degree 2 poles (36.803, 13.9135) (36.1773, 13.9135) (35.461, 14.766) (35.461, 15.4986) knots 0 0 0 1 2 2 2
  spline S40 degree 2 poles (35.461, 15.4986) (35.461, 16.2506) (36.2, 17.0837) (36.803, 17.0837) knots 0 0 0 1 2 2 2
  spline S41 degree 2 poles (36.803, 17.0837) (37.4124, 17.0837) (38.1417, 16.2539) (38.1417, 15.4986) knots 0 0 0 1 2 2 2
  spline S42 degree 2 poles (37.6198, 15.4986) (37.6198, 16.0821) (37.1952, 16.6493) (36.803, 16.6493) knots 0 0 0 1 2 2 2
  spline S43 degree 2 poles (36.803, 16.6493) (36.4107, 16.6493) (35.9829, 16.0821) (35.9829, 15.4986) knots 0 0 0 1 2 2 2
  spline S44 degree 2 poles (35.9829, 15.4986) (35.9829, 14.9314) (36.4107, 14.3479) (36.803, 14.3479) knots 0 0 0 1 2 2 2
  spline S45 degree 2 poles (36.803, 14.3479) (37.1919, 14.3479) (37.6198, 14.9216) (37.6198, 15.4986) knots 0 0 0 1 2 2 2
  line L42 (39.1757, 13.9978) -> (38.6701, 13.9978)
  line L43 (38.6701, 13.9978) -> (38.6701, 18.1761)
  line L44 (38.6701, 18.1761) -> (39.1757, 18.1761)
  line L45 (39.1757, 18.1761) -> (39.1757, 13.9978)
  line L46 (42.226, 13.9978) -> (41.7203, 13.9978)
  line L47 (41.7203, 13.9978) -> (41.7203, 14.3025)
  spline S46 degree 2 poles (41.7203, 14.3025) (41.6036, 14.2053) (41.4318, 14.0756) (41.3151, 14.0205) knots 0 0 0 1 2 2 2
  spline S47 degree 2 poles (41.3151, 14.0205) (41.2081, 13.9686) (40.978, 13.9135) (40.8256, 13.9135) knots 0 0 0 1 2 2 2
  spline S48 degree 2 poles (40.8256, 13.9135) (40.5793, 13.9135) (40.1644, 14.1177) (40.0185, 14.3155) knots 0 0 0 1 2 2 2
  spline S49 degree 2 poles (40.0185, 14.3155) (39.8726, 14.5132) (39.7106, 15.0967) (39.7106, 15.4759) knots 0 0 0 1 2 2 2
  spline S50 degree 2 poles (39.7106, 15.4759) (39.7106, 15.8714) (39.9148, 16.4484) (40.0931, 16.6656) knots 0 0 0 1 2 2 2
  spline S51 degree 2 poles (40.0931, 16.6656) (40.2584, 16.86) (40.7219, 17.0837) (40.978, 17.0837) knots 0 0 0 1 2 2 2
  spline S52 degree 2 poles (40.978, 17.0837) (41.2017, 17.0837) (41.5355, 16.9832) (41.7203, 16.8795) knots 0 0 0 1 2 2 2
  line L48 (41.7203, 16.8795) -> (41.7203, 18.1761)
  line L49 (41.7203, 18.1761) -> (42.226, 18.1761)
  line L50 (42.226, 18.1761) -> (42.226, 13.9978)
  line L51 (41.7203, 14.7271) -> (41.7203, 16.4613)
  spline S53 degree 2 poles (41.7203, 16.4613) (41.5323, 16.5521) (41.2341, 16.6202) (41.0623, 16.6202) knots 0 0 0 1 2 2 2
  spline S54 degree 2 poles (41.0623, 16.6202) (40.6733, 16.6202) (40.2325, 16.0367) (40.2325, 15.4857) knots 0 0 0 1 2 2 2
  spline S55 degree 2 poles (40.2325, 15.4857) (40.2325, 14.954) (40.5696, 14.3933) (40.9423, 14.3933) knots 0 0 0 1 2 2 2
  spline S56 degree 2 poles (40.9423, 14.3933) (41.1401, 14.3933) (41.542, 14.5748) (41.7203, 14.7271) knots 0 0 0 1 2 2 2
  spline S57 degree 2 poles (44.2616, 13.9297) (43.542, 13.9297) (42.7511, 14.7369) (42.7511, 15.4824) knots 0 0 0 1 2 2 2
  spline S58 degree 2 poles (42.7511, 15.4824) (42.7511, 16.215) (43.5193, 17.0837) (44.1384, 17.0837) knots 0 0 0 1 2 2 2
  spline S59 degree 2 poles (44.1384, 17.0837) (44.4172, 17.0837) (44.8483, 16.9216) (45.0072, 16.7498) knots 0 0 0 1 2 2 2
  spline S60 degree 2 poles (45.0072, 16.7498) (45.1692, 16.578) (45.341, 16.0821) (45.341, 15.7223) knots 0 0 0 1 2 2 2
  line L52 (45.341, 15.7223) -> (45.341, 15.4468)
  line L53 (45.341, 15.4468) -> (43.2632, 15.4468)
  spline S61 degree 2 poles (43.2632, 15.4468) (43.2632, 14.9249) (43.7884, 14.3706) (44.2551, 14.3706) knots 0 0 0 1 2 2 2
  spline S62 degree 2 poles (44.2551, 14.3706) (44.4205, 14.3706) (44.7414, 14.4451) (44.871, 14.5035) knots 0 0 0 1 2 2 2
  spline S63 degree 2 poles (44.871, 14.5035) (45.0072, 14.5683) (45.1952, 14.6818) (45.2568, 14.7336) knots 0 0 0 1 2 2 2
  line L54 (45.2568, 14.7336) -> (45.2859, 14.7336)
  line L55 (45.2859, 14.7336) -> (45.2859, 14.1826)
  spline S64 degree 2 poles (45.2859, 14.1826) (45.1984, 14.1469) (44.9326, 14.0432) (44.8289, 14.014) knots 0 0 0 1 2 2 2
  spline S65 degree 2 poles (44.8289, 14.014) (44.683, 13.9719) (44.4432, 13.9297) (44.2616, 13.9297) knots 0 0 0 1 2 2 2
  spline S66 degree 2 poles (44.8483, 15.8325) (44.8419, 16.0367) (44.7576, 16.3349) (44.6765, 16.4354) knots 0 0 0 1 2 2 2
  spline S67 degree 2 poles (44.6765, 16.4354) (44.589, 16.5489) (44.3135, 16.6688) (44.1093, 16.6688) knots 0 0 0 1 2 2 2
  spline S68 degree 2 poles (44.1093, 16.6688) (43.9083, 16.6688) (43.6263, 16.5489) (43.5096, 16.4322) knots 0 0 0 1 2 2 2
  spline S69 degree 2 poles (43.5096, 16.4322) (43.3961, 16.3122) (43.2795, 16.0237) (43.2632, 15.8325) knots 0 0 0 1 2 2 2
  line L56 (43.2632, 15.8325) -> (44.8483, 15.8325)
  line L57 (47.4448, 16.4581) -> (47.4188, 16.4581)
  spline S70 degree 2 poles (47.4188, 16.4581) (47.3605, 16.4743) (47.2341, 16.4808) (47.1466, 16.4808) knots 0 0 0 1 2 2 2
  spline S71 degree 2 poles (47.1466, 16.4808) (46.9423, 16.4808) (46.5404, 16.3025) (46.3589, 16.1275) knots 0 0 0 1 2 2 2
  line L58 (46.3589, 16.1275) -> (46.3589, 13.9978)
  line L59 (46.3589, 13.9978) -> (45.8532, 13.9978)
  line L60 (45.8532, 13.9978) -> (45.8532, 16.9994)
  line L61 (45.8532, 16.9994) -> (46.3589, 16.9994)
  line L62 (46.3589, 16.9994) -> (46.3589, 16.5521)
  spline S72 degree 2 poles (46.3589, 16.5521) (46.6344, 16.7985) (47.0461, 16.9994) (47.2406, 16.9994) knots 0 0 0 1 2 2 2
  spline S73 degree 2 poles (47.2406, 16.9994) (47.3184, 16.9994) (47.3961, 16.9929) (47.4448, 16.9832) knots 0 0 0 1 2 2 2
  line L63 (47.4448, 16.9832) -> (47.4448, 16.4581)
  line L64 (52.495, 17.9978) -> (51.1174, 13.9978)
  line L65 (51.1174, 13.9978) -> (50.5436, 13.9978)
  line L66 (50.5436, 13.9978) -> (49.166, 17.9978)
  line L67 (49.166, 17.9978) -> (49.7365, 17.9978)
  line L68 (49.7365, 17.9978) -> (50.8451, 14.6753)
  line L69 (50.8451, 14.6753) -> (51.9537, 17.9978)
  line L70 (51.9537, 17.9978) -> (52.495, 17.9978)
  line L71 (55.0299, 13.9978) -> (53.0785, 13.9978)
  line L72 (53.0785, 13.9978) -> (53.0785, 14.4062)
  line L73 (53.0785, 14.4062) -> (53.8046, 14.4062)
  line L74 (53.8046, 14.4062) -> (53.8046, 17.0869)
  line L75 (53.8046, 17.0869) -> (53.0785, 17.0869)
  line L76 (53.0785, 17.0869) -> (53.0785, 17.4532)
  spline S74 degree 2 poles (53.0785, 17.4532) (53.4902, 17.4532) (53.8791, 17.6866) (53.9051, 18.0108) knots 0 0 0 1 2 2 2
  line L77 (53.9051, 18.0108) -> (54.32, 18.0108)
  line L78 (54.32, 18.0108) -> (54.32, 14.4062)
  line L79 (54.32, 14.4062) -> (55.0299, 14.4062)
  line L80 (55.0299, 14.4062) -> (55.0299, 13.9978)
  line L81 (56.6247, 13.9978) -> (55.9829, 13.9978)
  line L82 (55.9829, 13.9978) -> (55.9829, 14.7628)
  line L83 (55.9829, 14.7628) -> (56.6247, 14.7628)
  line L84 (56.6247, 14.7628) -> (56.6247, 13.9978)
  spline S75 degree 2 poles (59.9213, 15.9978) (59.9213, 14.9216) (59.2957, 13.9135) (58.6441, 13.9135) knots 0 0 0 1 2 2 2
  spline S76 degree 2 poles (58.6441, 13.9135) (57.9829, 13.9135) (57.3637, 14.9411) (57.3637, 15.9946) knots 0 0 0 1 2 2 2
  spline S77 degree 2 poles (57.3637, 15.9946) (57.3637, 17.0772) (57.9893, 18.0788) (58.6441, 18.0788) knots 0 0 0 1 2 2 2
  spline S78 degree 2 poles (58.6441, 18.0788) (59.3021, 18.0788) (59.9213, 17.0416) (59.9213, 15.9978) knots 0 0 0 1 2 2 2
  spline S79 degree 2 poles (59.2341, 14.779) (59.3119, 14.9767) (59.3767, 15.5861) (59.3767, 15.9978) knots 0 0 0 1 2 2 2
  spline S80 degree 2 poles (59.3767, 15.9978) (59.3767, 16.4095) (59.3119, 17.0156) (59.2308, 17.2198) knots 0 0 0 1 2 2 2
  spline S81 degree 2 poles (59.2308, 17.2198) (59.1498, 17.4241) (58.8678, 17.6348) (58.6441, 17.6348) knots 0 0 0 1 2 2 2
  spline S82 degree 2 poles (58.6441, 17.6348) (58.4205, 17.6348) (58.132, 17.4241) (58.0477, 17.2134) knots 0 0 0 1 2 2 2
  spline S83 degree 2 poles (58.0477, 17.2134) (57.9667, 17.0092) (57.9083, 16.3868) (57.9083, 15.9946) knots 0 0 0 1 2 2 2
  spline S84 degree 2 poles (57.9083, 15.9946) (57.9083, 15.5732) (57.9602, 15.0092) (58.0444, 14.7887) knots 0 0 0 1 2 2 2
  spline S85 degree 2 poles (58.0444, 14.7887) (58.1222, 14.5813) (58.4107, 14.3576) (58.6441, 14.3576) knots 0 0 0 1 2 2 2
  spline S86 degree 2 poles (58.6441, 14.3576) (58.8645, 14.3576) (59.153, 14.5683) (59.2341, 14.779) knots 0 0 0 1 2 2 2
  spline S87 degree 2 poles (36.7008, 7.3276) (36.3475, 7.3276) (35.8224, 7.5124) (35.6376, 7.6972) knots 0 0 0 1 2 2 2
  spline S88 degree 2 poles (35.6376, 7.6972) (35.4269, 7.9046) (35.2551, 8.4881) (35.2551, 8.916) knots 0 0 0 1 2 2 2
  line L85 (35.2551, 8.916) -> (35.2551, 11.4119)
  line L86 (35.2551, 11.4119) -> (35.7867, 11.4119)
  line L87 (35.7867, 11.4119) -> (35.7867, 8.916)
  spline S89 degree 2 poles (35.7867, 8.916) (35.7867, 8.6372) (35.8581, 8.2612) (35.9585, 8.1088) knots 0 0 0 1 2 2 2
  spline S90 degree 2 poles (35.9585, 8.1088) (36.0655, 7.9468) (36.435, 7.7814) (36.7008, 7.7814) knots 0 0 0 1 2 2 2
  spline S91 degree 2 poles (36.7008, 7.7814) (36.9504, 7.7814) (37.3394, 7.9468) (37.4464, 8.1088) knots 0 0 0 1 2 2 2
  spline S92 degree 2 poles (37.4464, 8.1088) (37.5469, 8.2612) (37.6182, 8.634) (37.6182, 8.903) knots 0 0 0 1 2 2 2
  line L88 (37.6182, 8.903) -> (37.6182, 11.4119)
  line L89 (37.6182, 11.4119) -> (38.1498, 11.4119)
  line L90 (38.1498, 11.4119) -> (38.1498, 8.916)
  spline S93 degree 2 poles (38.1498, 8.916) (38.1498, 8.4978) (37.9812, 7.9014) (37.7673, 7.6972) knots 0 0 0 1 2 2 2
  spline S94 degree 2 poles (37.7673, 7.6972) (37.5761, 7.5092) (37.0704, 7.3276) (36.7008, 7.3276) knots 0 0 0 1 2 2 2
  spline S95 degree 2 poles (40.4739, 7.3406) (40.085, 7.3406) (39.4269, 7.6032) (39.1871, 7.8657) knots 0 0 0 1 2 2 2
  spline S96 degree 2 poles (39.1871, 7.8657) (38.9472, 8.125) (38.6846, 8.903) (38.6846, 9.4087) knots 0 0 0 1 2 2 2
  spline S97 degree 2 poles (38.6846, 9.4087) (38.6846, 9.9111) (38.9407, 10.6566) (39.1838, 10.9322) knots 0 0 0 1 2 2 2
  spline S98 degree 2 poles (39.1838, 10.9322) (39.4237, 11.2012) (40.0785, 11.4832) (40.4837, 11.4832) knots 0 0 0 1 2 2 2
  spline S99 degree 2 poles (40.4837, 11.4832) (40.6846, 11.4832) (41.038, 11.4249) (41.1871, 11.3795) knots 0 0 0 1 2 2 2
  spline S100 degree 2 poles (41.1871, 11.3795) (41.3167, 11.3374) (41.5858, 11.2174) (41.7187, 11.1461) knots 0 0 0 1 2 2 2
  line L91 (41.7187, 11.1461) -> (41.7187, 10.5043)
  line L92 (41.7187, 10.5043) -> (41.6765, 10.5043)
  spline S101 degree 2 poles (41.6765, 10.5043) (41.6052, 10.5691) (41.3848, 10.7506) (41.226, 10.8382) knots 0 0 0 1 2 2 2
  spline S102 degree 2 poles (41.226, 10.8382) (41.0736, 10.9224) (40.7138, 11.0294) (40.4804, 11.0294) knots 0 0 0 1 2 2 2
  spline S103 degree 2 poles (40.4804, 11.0294) (40.2243, 11.0294) (39.7673, 10.8187) (39.5955, 10.6177) knots 0 0 0 1 2 2 2
  spline S104 degree 2 poles (39.5955, 10.6177) (39.4269, 10.4135) (39.2389, 9.7944) (39.2389, 9.4087) knots 0 0 0 1 2 2 2
  spline S105 degree 2 poles (39.2389, 9.4087) (39.2389, 8.997) (39.4367, 8.4038) (39.6085, 8.1996) knots 0 0 0 1 2 2 2
  spline S106 degree 2 poles (39.6085, 8.1996) (39.777, 8.0019) (40.2276, 7.8009) (40.4804, 7.8009) knots 0 0 0 1 2 2 2
  spline S107 degree 2 poles (40.4804, 7.8009) (40.7106, 7.8009) (41.1028, 7.9143) (41.2551, 7.9986) knots 0 0 0 1 2 2 2
  spline S108 degree 2 poles (41.2551, 7.9986) (41.401, 8.0829) (41.6182, 8.2579) (41.6798, 8.3195) knots 0 0 0 1 2 2 2
  line L93 (41.6798, 8.3195) -> (41.7187, 8.3195)
  line L94 (41.7187, 8.3195) -> (41.7187, 7.6842)
  spline S109 degree 2 poles (41.7187, 7.6842) (41.5858, 7.6226) (41.3524, 7.5092) (41.1871, 7.4573) knots 0 0 0 1 2 2 2
  spline S110 degree 2 poles (41.1871, 7.4573) (41.012, 7.3989) (40.7138, 7.3406) (40.4739, 7.3406) knots 0 0 0 1 2 2 2
  spline S111 degree 2 poles (45.3686, 9.4087) (45.3686, 8.8609) (44.9245, 7.9792) (44.5517, 7.7328) knots 0 0 0 1 2 2 2
  spline S112 degree 2 poles (44.5517, 7.7328) (44.247, 7.5416) (43.6214, 7.4119) (43.1352, 7.4119) knots 0 0 0 1 2 2 2
  line L95 (43.1352, 7.4119) -> (42.2146, 7.4119)
  line L96 (42.2146, 7.4119) -> (42.2146, 11.4119)
  line L97 (42.2146, 11.4119) -> (43.1255, 11.4119)
  spline S113 degree 2 poles (43.1255, 11.4119) (43.6895, 11.4119) (44.3313, 11.2434) (44.5582, 11.0942) knots 0 0 0 1 2 2 2
  spline S114 degree 2 poles (44.5582, 11.0942) (44.944, 10.8382) (45.3686, 9.9921) (45.3686, 9.4087) knots 0 0 0 1 2 2 2
  spline S115 degree 2 poles (44.8143, 9.4152) (44.8143, 9.8754) (44.5096, 10.527) (44.2081, 10.7118) knots 0 0 0 1 2 2 2
  spline S116 degree 2 poles (44.2081, 10.7118) (43.9942, 10.8382) (43.5112, 10.9516) (43.1514, 10.9516) knots 0 0 0 1 2 2 2
  line L98 (43.1514, 10.9516) -> (42.7462, 10.9516)
  line L99 (42.7462, 10.9516) -> (42.7462, 7.8722)
  line L100 (42.7462, 7.8722) -> (43.1514, 7.8722)
  spline S117 degree 2 poles (43.1514, 7.8722) (43.5047, 7.8722) (44.0396, 7.9857) (44.2568, 8.138) knots 0 0 0 1 2 2 2
  spline S118 degree 2 poles (44.2568, 8.138) (44.5355, 8.326) (44.8143, 8.9484) (44.8143, 9.4152) knots 0 0 0 1 2 2 2
  point P0 (0, 0)
  constraints: 2 other
emboss "Emboss2" sketch "Sketch4" operation cut depth 5 direction (0, -1, 0) contours S0 S1 L8 L9 L10 L11 L12 S2 S3 | S8 S9 S10 S11 S12 S13 L16 L17 S14 S15 S16 S17 S18 S19 S20 S21 L18 L19 S22 S23 | S24 S25 L20 L21 L22 S26 S27 S28 L23 S29 | L30 L31 L32 L33 L34 L35 L36 L37 L38 L39 L40 L41 | S38 S39 S40 S41 | L42 L43 L44 L45 | L46 L47 S46 S47 S48 S49 S50 S51 S52 L48 L49 L50 | S57 S58 S59 S60 L52 L53 S61 S62 S63 L54 L55 S64 S65 | L57 S70 S71 L58 L59 L60 L61 L62 S72 S73 L63 | L64 L65 L66 L67 L68 L69 L70 | L71 L72 L73 L74 L75 L76 S74 L77 L78 L79 L80 | L81 L82 L83 L84 | S75 S76 S77 S78 | S87 S88 L85 L86 L87 S89 S90 S91 S92 L88 L89 L90 S93 S94 | S95 S96 S97 S98 S99 S100 L91 L92 S101 S102 S103 S104 S105 S106 S107 S108 L93 L94 S109 S110 | S111 S112 L95 L96 L97 S113 S114
sketch "Sketch5" plane through (80, 0, 0) normal (1, 0, 0) x (0, 0, -1)
  line L0 (160, 0) -> (160, 28) projected
  line L1 (0, 0) -> (160, 0)
  line L2 (160, 0) -> (160, 15)
  line L3 (160, 15) -> (0, 15)
  line L4 (0, 15) -> (0, 0)
  line L5 (49.2749, 5) -> (44.8614, 5) projected
  point P0 (47.0682, 5)
  dimension "d46" = 10
  constraints: 8 end point, 2 parallel, 1 horizontal, 1 midpoint, 1 perpendicular, 1 point on line
  measures "d46" distance from line of point (47.068, 5) L3
extrude "Extrusion3" add sketch "Sketch5" against normal blind 5
ref_plane "Work Plane1" through (40, 0, 0) normal (1, 0, 0) x (0, 0, -1)
mirror "Mirror1" about plane through (40, 0, 0) normal (1, 0, 0) of "Extrusion3"
equation "\"d25\" = d23"
equation "\"d26\" = d23"
equation "\"d27\" = d23"
equation "\"d28\" = d23"
equation "\"d29\" = d23"
equation "\"d30\" = d23"
equation "\"d31\" = d24"
equation "\"d32\" = d24"
equation "\"d33\" = d24"
equation "\"d34\" = d24"
equation "\"d35\" = d24"
equation "\"d36\" = d24"
equation "\"d37\" = d24"
equation "\"d42\" = d23"
equation "\"d43\" = d24"
body "Solid1"
